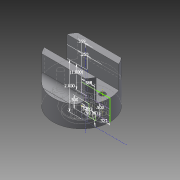
# Autodesk Inventor part: denso-1in-square-tube coupler rev2
Saved by Autodesk Inventor 2015 (Build 190159000, 159)
## iProperties
Created: 2015-02-04
Part Number: denso-1in-square-tube coupler rev2
Material: Generic
Document SubType Name: Modeling
Designer: sethbattis
Density: 1 g/cm^3
Appearance: Default
Author: sethbattis
Autodesk Inventor part; units mm, degrees
ref_plane "YZ Plane" through (0, 0, 0) normal (1, 0, 0) x (0, 1, 0)
ref_plane "XZ Plane" through (0, 0, 0) normal (0, 1, 0) x (-1, 0, 0)
ref_plane "XY Plane" through (0, 0, 0) normal (0, 0, 1) x (1, 0, 0)
sketch "Sketch1" plane through (0, 0, 0) normal (0, 0, 1) x (1, 0, 0)
  line L0 (0, 0) -> (0, 50.8) construction
  line L1 (0, 0) -> (50.8, 0) construction
  line L2 (0, 50.8) -> (6.35, 50.8) construction
  line L3 (6.35, 50.8) -> (6.35, 0) construction
  line L4 (0, 25.4) -> (14.9225, 25.4) construction
  line L5 (31.75, 12.7) -> (31.75, 25.4)
  line L6 (14.9225, 25.4) -> (31.75, 25.4)
  line L7 (0, 9.5479) -> (15.8115, 9.5479) construction
  line L8 (31.75, 12.7) -> (15.875, 12.7)
  line L9 (15.875, 12.7) -> (15.875, 6.2992)
  line L10 (0, 19.05) -> (31.75, 19.05) construction
  line L11 (0, 6.2992) -> (8.2867, 6.2992) construction
  line L12 (8.2867, 6.2992) -> (15.875, 6.2992)
  line L13 (8.2867, 6.2992) -> (8.2867, 18.9992)
  line L14 (23.5585, 11.9908) -> (23.5585, 41.3472) construction
  line L15 (4.0259, 71.0633) -> (4.0259, -11.3243) construction
  line L16 (8.2867, 18.9992) -> (4.0259, 18.9992)
  line L17 (4.0259, 25.4) -> (6.35, 25.4)
  line L18 (4.0259, 25.4) -> (4.0259, 18.9992)
  line L19 (31.75, 36.068) -> (31.75, 25.4)
  line L20 (31.75, 36.068) -> (0, 36.068)
  line L21 (4.0259, 25.4) -> (0, 25.4)
  line L22 (0, 36.068) -> (0, 25.4)
  dimension "d2" = 50.8
  dimension "d3" = 90
  dimension "d4" = 6.35
  dimension "d6" = 14.9225
  dimension "d12" = 15.8115
  dimension "d15" = 8.2867
  dimension "d28" = 8.1915
  dimension "d55" = 4.0259
  dimension "d56" = 12.7
  dimension "d57" = 25.4
  dimension "d73" = 12.7
  constraints: 47 end point, 8 perpendicular, 8 point on line, 5 horizontal, 4 midpoint, 4 vertical, 3 collinear, 1 horizontal alignment, 1 parallel
  measures "d2" distance of L0.start L0.end
  measures "d3" angle of L1 L0
  measures "d4" distance of L0.end L2.end
  measures "d6" distance of L4.start L4.end
  measures "d12" distance of L7.start L7.end
  measures "d15" distance of L11.start L11.end
  measures "d28" distance between parallel lines of L5 L14
  measures "d55" distance between parallel lines of L0 L15
  measures "d56" distance of L11.end L13.end
  measures "d57" distance of L2.end L17.end
  measures "d73" distance between parallel lines of L6 L8
revolve "Revolution1" add sketch "Sketch1" angle 360 about axis through (0, 0, 0) along (0, 1, 0)
fillet "Fillet2" radius 2.921 1 edges at (-15.875, 12.7, 0)
hole "Hole2" at (23.5947, 36.068, 0.0381) direction (0, -1, 0) diameter 6.35 end through all
pattern_circular "Circular Pattern1" count 2 over 360 about axis through (0, 22.1996, 0) along (0, -1, 0) of "Hole2"
sketch "Sketch2" plane through (0, 6.2992, 0) normal (0, -1, 0) x (1, 0, 0)
  circle A0 centre (0, 0) radius 8.2867 construction
  line L0 (-2.2055, 7.9879) -> (-2.2121, 9.8928)
  circle A1 centre (0, 0) radius 10.1371 construction
  line L1 (2.1506, 8.0028) -> (2.144, 9.9078)
  line L2 (-2.2055, 7.9879) -> (2.1506, 8.0028) construction
  arc A2 (2.144, 9.9078) -> (-2.2121, 9.8928) centre (0, 0) ccw
  arc A3 (2.1506, 8.0028) -> (-2.2055, 7.9879) centre (0, 0) ccw
  dimension "d43" = 1.905
  dimension "d44" = 4.3561
  constraints: 8 point on circle, 6 end point, 3 centre point, 2 coincident, 1 concentric, 1 parallel, 1 perpendicular
  measures "d43" distance of L0.start L0.end
  measures "d44" distance of L0.start L1.start
extrude "Extrusion1" cut sketch "Sketch2" against normal blind 12.7
pattern_circular "Circular Pattern2" count 6 over 360 about axis through (0, 12.6492, 0) along (0, -1, 0) of "Extrusion1"
sketch "Sketch5" plane through (0, 12.7, 0) normal (0, -1, 0) x (1, 0, 0)
  point P0 (0, 0)
sketch "Sketch6" plane through (0, 12.7, 0) normal (0, -1, 0) x (1, 0, 0)
  circle A0 centre (23.5947, 0.0381) radius 6.4135 construction
  circle A1 centre (23.5947, 0.0381) radius 3.175 construction
  line L0 (29.149, 3.2449) -> (29.149, -3.1686)
  line L1 (29.149, -3.1686) -> (23.5947, -6.3754)
  line L2 (23.5947, -6.3754) -> (18.0405, -3.1686)
  line L3 (18.0405, -3.1686) -> (18.0405, 3.2449)
  line L4 (18.0405, 3.2449) -> (23.5947, 6.4516)
  line L5 (23.5947, 6.4516) -> (29.149, 3.2449)
  point P0 (0, 0)
  dimension "d74" = 12.827
  constraints: 12 end point, 5 equal length, 5 point on circle, 1 centre point, 1 coincident, 1 concentric, 1 parallel, 1 vertical
  measures "d74" diameter of A0
extrude "Extrusion4" cut sketch "Sketch6" along normal mid plane 8.6868
pattern_circular "Circular Pattern3" count 2 over 360 about axis through (0, 9.779, 0) along (0, -1, 0) of "Extrusion4"
sketch "Sketch7" plane through (0, 36.068, 0) normal (0, 1, 0) x (1, 0, 0)
  circle A0 centre (0, 0) radius 31.75 construction
  line L0 (-31.75, 0) -> (31.75, 0) construction
  line L1 (-29.0994, 12.7) -> (29.0994, 12.7)
  line L2 (-29.0994, -12.7) -> (29.0994, -12.7)
  line L3 (-24.3959, 20.32) -> (24.3959, 20.32)
  line L4 (-24.3959, -20.32) -> (24.3959, -20.32)
  arc A1 (-29.0994, -12.7) -> (-24.3959, -20.32) centre (0, 0) ccw
  arc A2 (24.3959, -20.32) -> (29.0994, -12.7) centre (0, 0) ccw
  arc A3 (29.0994, 12.7) -> (24.3959, 20.32) centre (0, 0) ccw
  arc A4 (-24.3959, 20.32) -> (-29.0994, 12.7) centre (0, 0) ccw
  dimension "d94" = 63.5
  dimension "d88" = 25.4
  dimension "d89" = 7.62
  dimension "d90" = 7.62
  constraints: 10 end point, 8 point on circle, 5 horizontal, 4 centre point, 1 midpoint, 13 other
  measures "d88" distance between parallel lines of L1 L2
  measures "d89" distance between parallel lines of L2 L4
  measures "d90" distance between parallel lines of L3 L1
extrude "Extrusion5" add sketch "Sketch7" along normal blind 25.4
fillet "Fillet7" radius 7.62 2 edges at (0, 36.068, 20.32) (0, 36.068, -20.32)
equation "\"d90\" = d89"
body "Solid1"
